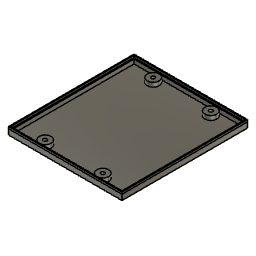
VersaTermBottom (Autodesk Fusion 360 design; units mm, degrees)
Autodesk Fusion 360 part; units mm, degrees
box "BoxPrimitive1" add length 104.5 width 94.5 height 5.5 placed x (0, 1, 0) y (-1, 0, 0) z (0, 0, 1) at (94.5, 0, 0) makes body 1
shell "Shell1" thickness 2 removed faces 1 at (31.5, 34.8333, 5.5) on bodies 1
sketch "Sketch3" plane through (0, 0, 2) normal (0, 0, 1) x (-1, 0, 0)
  line L0 (-92.5, -102.5) -> (-2, -102.5)
  line L1 (-2, -102.5) -> (-2, -2)
  line L2 (-2, -2) -> (-92.5, -2)
  line L3 (-92.5, -2) -> (-92.5, -102.5)
  circle A0 centre (-23.25, -97.25) radius 5
  dimension "d7" = 10
  dimension "d8" = 5.25
  dimension "d9" = 21.25
  measures "d7" diameter of A0
  measures "d8" distance of L0 A0.centre
  measures "d9" distance of L1 A0.centre
extrude "Extrude1" add sketch "Sketch3" along normal blind 3.5 contours A0 bodies 1
sketch "Sketch6" plane through (0, 0, 0) normal (0, 0, -1) x (1, 0, 0)
  line L0 (0, -104.5) -> (94.5, -104.5)
  line L1 (94.5, -104.5) -> (94.5, 0)
  line L2 (94.5, 0) -> (0, 0)
  line L3 (0, 0) -> (0, -104.5)
  line L4 (19.4972, -97.25) -> (21.3736, -100.5)
  line L5 (21.3736, -100.5) -> (25.1264, -100.5)
  line L6 (25.1264, -100.5) -> (27.0028, -97.25)
  line L7 (27.0028, -97.25) -> (25.1264, -94)
  line L8 (25.1264, -94) -> (21.3736, -94)
  line L9 (21.3736, -94) -> (19.4972, -97.25)
  point P0 (23.25, -97.25)
  dimension "d12" = 3.25
  dimension "d13" = 23.25
  dimension "d14" = 7.25
  constraint horizontal L5
  measures "d12" distance of P0 L4
  measures "d13" distance of L3 P0
  measures "d14" distance of L0 P0
extrude "Extrude2" cut sketch "Sketch6" against normal blind 3.5 contours L4 L5 L6 L7 L8 L9 bodies 1
sketch "Sketch9" plane through (0, 0, 5.5) normal (0, 0, 1) x (-1, 0, 0)
  circle A0 centre (-23.25, -97.25) radius 5
  circle A1 centre (-23.25, -97.25) radius 1.55
  dimension "d18" = 3.1
  constraint concentric A0 A1
  measures "d18" diameter of A1
extrude "Extrude3" cut sketch "Sketch9" against normal blind 5 contours A1 bodies 1
pattern_linear "R-Pattern1" count 2 spacing 48 along (1, 0, 0) count 2 spacing 90 along (0, -1, 0) of "Extrude1", "Extrude2", "Extrude3"
sketch "Sketch12" plane through (0, 0, 5.5) normal (0, 0, 1) x (-1, 0, 0)
  line L0 (-92.5, -102.5) -> (-92.5, -2)
  line L1 (-92.5, -2) -> (-2, -2)
  line L2 (-2, -2) -> (-2, -102.5)
  line L3 (-2, -102.5) -> (-92.5, -102.5)
  line L4 (-94.5, -104.5) -> (0, -104.5)
  line L5 (0, -104.5) -> (0, 0)
  line L6 (0, 0) -> (-94.5, 0)
  line L7 (-94.5, 0) -> (-94.5, -104.5)
  line L8 (0, -104.5) -> (-94.5, -104.5)
  line L9 (-94.5, -104.5) -> (-94.5, 0)
  line L10 (-94.5, 0) -> (0, 0)
  line L11 (0, 0) -> (0, -104.5)
  line L12 (-0.9, -0.9) -> (-0.9, -103.6)
  line L13 (-0.9, -103.6) -> (-93.6, -103.6)
  line L14 (-93.6, -103.6) -> (-93.6, -0.9)
  line L15 (-93.6, -0.9) -> (-0.9, -0.9)
  dimension "d26" = 0.9
  constraint horizontal L8
  constraint vertical L9
  constraint horizontal L10
  constraint vertical L11
  constraint coincident L6.end L7.start
  constraint coincident L4.end L5.start
extrude "Extrude4" add sketch "Sketch12" along normal blind 1.6 separate body contours L4 L5 L6 L7 L8 L9 L10 L11 makes body 2
chamfer "Chamfer1" distance 1 angle 45 4 edges at (47.25, 104.5, 0) (0, 52.25, 0) (94.5, 52.25, 0) (47.25, 0, 0) on bodies 1
sketch "Sketch15" plane through (0, 0, 0) normal (-1, 0, 0) x (0, -1, 0)
  line L0 (-104.5, 1) -> (0, 1)
  line L1 (0, 1) -> (0, 5.5)
  line L2 (0, 5.5) -> (-104.5, 5.5)
  line L3 (-104.5, 5.5) -> (-104.5, 1)
  line L4 (-99.746, 5.5) -> (-68.186, 5.5)
  line L5 (-68.186, 5.5) -> (-68.186, 1)
  line L6 (-68.186, 1) -> (-99.746, 1)
  line L7 (-99.746, 1) -> (-99.746, 5.5)
  dimension "d30" = 31.56
  dimension "d31" = 4.754
  dimension "d34" = 4.5
  constraint horizontal L4
  constraint vertical L5
  constraint horizontal L6
  constraint vertical L7
  constraint coincident L0 L5.end
  measures "d30" distance of L5 L7
  measures "d31" distance of L3 L7
  measures "d34" distance of L4 L6
extrude "Extrude5" [rolled back] along distance 1.1 taper angle 0
sketch "Sketch17" plane through (0, 0, 0) normal (-1, 0, 0) x (0, -1, 0)
  line L0 (-99.746, 1) -> (-99.746, 5.5)
  line L1 (-99.746, 5.5) -> (-68.186, 5.5)
  line L2 (-68.186, 5.5) -> (-68.186, 1)
  line L3 (-68.186, 1) -> (0, 1)
  line L4 (0, 1) -> (0, 7.1)
  line L5 (0, 7.1) -> (-104.5, 7.1)
  line L6 (-104.5, 7.1) -> (-104.5, 1)
  line L7 (-104.5, 1) -> (-99.746, 1)
  line L8 (-99.746, 5.5) -> (-68.186, 5.5)
  line L9 (-68.186, 5.5) -> (-68.186, 7.1)
  line L10 (-68.186, 7.1) -> (-99.746, 7.1)
  line L11 (-99.746, 7.1) -> (-99.746, 5.5)
  constraint horizontal L8
  constraint vertical L9
  constraint horizontal L10
  constraint vertical L11
  constraint coincident L5 L9.end
  constraint coincident L0.end L1.start
  constraint collinear L2 L9
extrude "Extrude6" [rolled back] along distance 1.1 taper angle 0
draft "Draft1" [rolled back] angle1 -10.22 angle2 0
loft "Loft3" [rolled back]
sketch "Sketch19" plane through (0, 0, 0) normal (-1, 0, 0) x (0, -1, 0)
  line L0 (-68.186, 7.1) -> (-68.186, 1)
  line L1 (-68.186, 1) -> (0, 1)
  line L2 (0, 1) -> (0, 7.1)
  line L3 (0, 7.1) -> (-68.186, 7.1)
  line L4 (-68.186, 7.1) -> (-64, 7.1)
  line L5 (-64, 7.1) -> (-64, 1)
  line L6 (-64, 1) -> (-68.186, 1)
  line L7 (-68.186, 1) -> (-68.186, 7.1)
  dimension "d42" = 4.186
  constraint horizontal L4
  constraint vertical L5
  constraint horizontal L6
  constraint vertical L7
  constraint coincident L1 L5.end
  constraint coincident L0.start L3.end
  measures "d42" distance of L5 L7
loft "Loft4" [rolled back]
